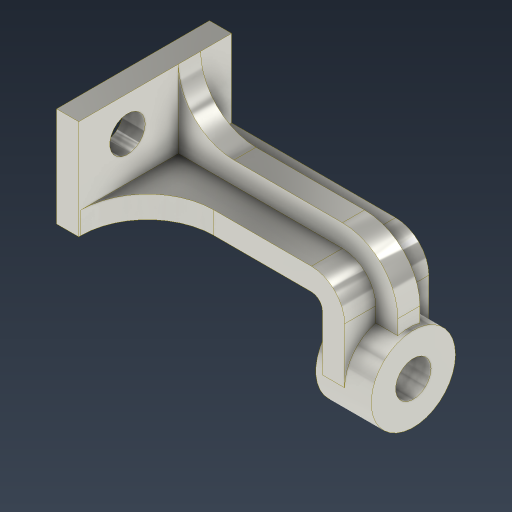
# Autodesk Inventor part: Peça teste 5
Saved by Autodesk Inventor 2024 (Build 280153000, 153)
## iProperties
Created: 2024-02-12
Part Number: Peça teste 5
Material: Prata
Document SubType Name: Modeling
Designer: Administrator
Density: 10.49 g/cm^3
Appearance: Prata
Author: Administrator
Autodesk Inventor part; units mm, degrees
ref_plane "YZ Plane" through (0, 0, 0) normal (1, 0, 0) x (0, 1, 0)
ref_plane "XZ Plane" through (0, 0, 0) normal (0, 1, 0) x (-1, 0, 0)
sketch "Esboço1" plane through (0, 0, 0) normal (1, 0, 0) x (0, 1, 0)
  line L0 (0, 0) -> (45, 0)
  line L1 (45, 0) -> (45, -69)
  line L2 (45, -69) -> (0, -69)
  line L3 (0, -69) -> (0, 0)
  dimension "d0" = 45
  dimension "d1" = 69
  constraints: 8 end point, 2 parallel, 1 horizontal, 1 perpendicular
  measures "d0" distance of L1.end L2.end
  measures "d1" distance of L0.end L1.end
extrude "Extrusão1" add sketch "Esboço1" along normal blind 10
sketch "Esboço2" plane through (10, 0, 0) normal (1, 0, 0) x (0, 0, -1)
  line L0 (0, 45) -> (0, 0) projected
  point P0 (22, 29.1579)
  dimension "d4" = 22
  measures "d4" distance from line of L0 point (22, 29.158)
hole "Furo1" at (10, 29.1579, -22) direction (-1, 0, 0) diameter 16 end through all
ref_plane "Plano de trabalho1" through (111, 0, 0) normal (1, 0, 0) x (0, 0, -1)
sketch "Esboço3" plane through (111, 0, 0) normal (1, 0, 0) x (0, 0, -1)
  circle A0 centre (50, -30) radius 19
  line L0 (69, 0) -> (69, 45) projected
  line L1 (69, 45) -> (0, 45) projected
  point P0 (0, 0)
  dimension "d13" = 38
  dimension "d14" = 75
  constraints: 1 centre point, 1 tangent
  measures "d13" diameter of A0
  measures "d14" distance from line of A0.centre L1
extrude "Extrusão2" add sketch "Esboço3" against normal blind 25
sketch "Esboço4" plane through (0, 0, -69) normal (0, 0, -1) x (-1, 0, 0)
  line L0 (-10, 0) -> (-84, 0)
  line L1 (-89, -5) -> (-89, -30)
  line L2 (-89, -30) -> (-99, -30)
  line L3 (-99, -30) -> (-99, -5)
  line L4 (-84, 10) -> (-10, 10)
  line L5 (-10, 10) -> (-10, 0)
  line L6 (-111, -11) -> (-111, -49) construction
  line L7 (-111, -30) -> (-86, -30) construction
  line L8 (-86, -49) -> (-86, -11) construction
  arc A0 (-84, 0) -> (-89, -5) centre (-84, -5) ccw
  arc A1 (-84, 10) -> (-99, -5) centre (-84, -5) ccw
  point P0 (0, 0)
  dimension "d17" = 3
  dimension "d18" = 10
  dimension "d19" = 10
  dimension "d20" = 5
  dimension "d21" = 15
  constraints: 14 end point, 5 perpendicular, 4 point on circle, 4 tangent, 2 centre point, 2 midpoint, 1 horizontal, 1 point on line
  measures "d17" distance between parallel lines of L8 L1
  measures "d18" distance between parallel lines of L1 L3
  measures "d19" distance between parallel lines of L0 L4
  measures "d20" radius of A0
  measures "d21" radius of A1
extrude "Extrusão3" add sketch "Esboço4" against normal blind 38
sketch "Esboço5" plane through (10, 0, 0) normal (1, 0, 0) x (0, 0, -1)
  line L0 (69, 10) -> (31, 10) projected
  line L1 (45, 10) -> (55, 10)
  line L2 (55, 10) -> (55, 20)
  line L3 (55, 20) -> (45, 20)
  line L4 (45, 20) -> (45, 10)
  line L5 (31, 10) -> (31, -5) projected
  point P0 (0, 0)
  dimension "d24" = 10
  dimension "d25" = 10
  dimension "d26" = 14
  constraints: 8 end point, 2 parallel, 1 horizontal, 1 perpendicular, 1 point on line
  measures "d24" distance of L3.end L2.end
  measures "d25" distance of L2.end L1.end
  measures "d26" distance between parallel lines of L4 L5
sketch3d "Esboço 3D1"
  line L0 (10, 10, -69) -> (84, 10, -69)
  arc A0 (84, 10, -69) -> (99, -5, -69) centre (84, -5, -69) ccw
  line L1 (99, -5, -69) -> (99, -30, -69)
sweep "Varredura1" add profiles "Esboço5" path "Esboço 3D1"
fillet "Arredondamento1" radius 25 1 edges at (10, 20, -50)
fillet "Arredondamento2" radius 30 1 edges at (10, 5, -31)
sketch "Esboço6" plane through (111, -30, -50) normal (1, 0, 0) x (0, 0, -1)
  circle A0 centre (0, 0) radius 19 projected
  point P0 (-50, 30)
  constraints: 1 coincident
hole "Furo2" at (111, -30, -50) direction (-1, 0, 0) diameter 16 end through all
